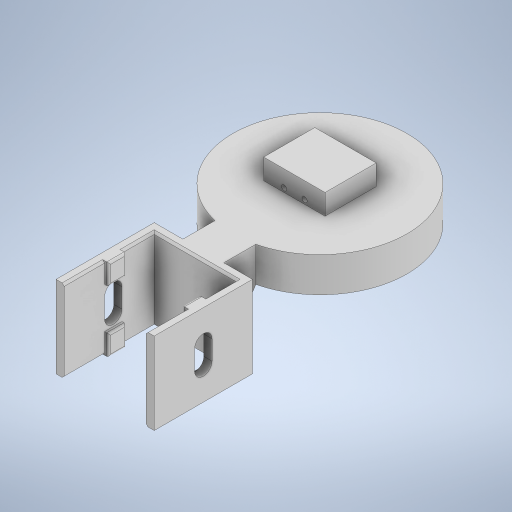
# Autodesk Inventor part: Bi_PAM_top_slot2
Saved by Autodesk Inventor 2024 (Build 280153000, 153)
## iProperties
Created: 2023-07-27
Part Number: Bi_PAM_top_slot2
Material: 일반
Document SubType Name: Modeling
Designer: jsw
Density: 1 g/cm^3
Appearance: 기본값
Author: jsw
Autodesk Inventor part; units mm, degrees
ref_plane "YZ Plane" through (0, 0, 0) normal (1, 0, 0) x (0, 1, 0)
ref_plane "XZ Plane" through (0, 0, 0) normal (0, 1, 0) x (-1, 0, 0)
sketch "스케치1" plane through (0, 0, 0) normal (0, 1, 0) x (-1, 0, 0)
  circle A0 centre (0, 0) radius 39
  circle A1 centre (0, 0) radius 42.5
  dimension "d0" = 78
  dimension "d1" = 3.5
  constraints: 2 centre point, 2 coincident
  measures "d0" diameter of A0
  measures "d1" radial gap between concentric circles of A0 A1
extrude "돌출1" add sketch "스케치1" along normal blind 7 contours A0 | A1
sketch "스케치2" plane through (0, 0, 0) normal (0, -1, 0) x (1, 0, 0)
  line L0 (15, -36.2132) -> (-15, -36.2132)
  line L1 (-15, -36.2132) -> (-36.2132, -15)
  line L2 (-36.2132, -15) -> (-36.2132, 15)
  line L3 (-36.2132, 15) -> (-15, 36.2132)
  line L4 (-15, 36.2132) -> (15, 36.2132)
  line L5 (15, 36.2132) -> (36.2132, 15)
  line L6 (36.2132, 15) -> (36.2132, -15)
  line L7 (36.2132, -15) -> (15, -36.2132)
  point P0 (0, 0)
  point P1 (0, 0)
  dimension "d5" = 30
  constraints: 16 end point, 1 coincident, 1 horizontal, 17 other
  measures "d5" distance of L5.end L6.end
extrude "돌출2" cut sketch "스케치2" against normal blind 4
fillet "모깎기1" radius 1.2 8 edges at (0, 4, 36.2132) (-25.6066, 4, 25.6066) (25.6066, 4, 25.6066) (36.2132, 4, 0) (25.6066, 4, -25.6066) (0, 4, -36.2132) (-25.6066, 4, -25.6066) (-36.2132, 4, 0)
sketch "스케치3" plane through (0, 0, 0) normal (0, -1, 0) x (1, 0, 0)
  line L0 (-15, 36.2132) -> (15, 36.2132) projected
  circle A0 centre (0, 0) radius 39.1969
  circle A1 centre (0, 0) radius 41.1969
  dimension "d9" = 2
  constraints: 2 coincident, 1 centre point, 3 other
extrude "돌출3" cut sketch "스케치3" against normal blind 4
sketch "스케치4" plane through (0, 7, 0) normal (0, 1, 0) x (1, 0, 0)
  line L0 (-15, 12.5) -> (15, 12.5)
  line L1 (15, 12.5) -> (15, -12.5)
  line L2 (15, -12.5) -> (-15, -12.5)
  line L3 (-15, -12.5) -> (-15, 12.5)
  point P0 (0, 0)
  point P1 (0, 12.5)
  point P2 (15, 0)
  dimension "d12" = 30
  dimension "d13" = 25
  constraints: 8 end point, 2 midpoint, 2 parallel, 1 horizontal, 1 horizontal alignment, 1 perpendicular, 1 vertical alignment
  measures "d12" distance of L0.start L0.end
  measures "d13" distance of L0.end L1.end
extrude "돌출4" add sketch "스케치4" along normal blind 10
sketch "스케치10" plane through (0, 0, 0) normal (0, -1, 0) x (1, 0, 0)
  circle A0 centre (0, 0) radius 41.1969 projected
  circle A1 centre (0, 0) radius 42.5 projected
extrude "돌출9" add sketch "스케치10" along normal blind 10
sketch "스케치11" plane through (0, 7, 0) normal (0, 1, 0) x (1, 0, 0)
  line L0 (-10, -61) -> (10, -61)
  line L1 (10, -61) -> (10, -41)
  line L2 (10, -41) -> (-10, -41)
  line L3 (-10, -41) -> (-10, -61)
  line L4 (-10, -61) -> (10, -41) construction
  line L5 (10, -61) -> (-10, -41) construction
  circle A0 centre (0, 0) radius 42.5 projected
  point P0 (0, -51)
  point P1 (10, -41.3068)
  point P2 (-10, -41.3068)
  dimension "d44" = 10
  dimension "d45" = 20
  dimension "d49" = 41
  constraints: 12 end point, 2 midpoint, 2 parallel, 1 horizontal, 1 perpendicular, 1 vertical alignment
  measures "d44" distance from line of point (0, -51) L1
  measures "d45" distance of L0.end L1.end
  measures "d49" distance from line of L2 point (0, 0)
extrude "돌출10" add sketch "스케치11" against normal blind 40 contours L3 A0 L1 L0
sketch "스케치12" plane through (0, 7, 0) normal (0, 1, 0) x (1, 0, 0)
  line L0 (20, -101) -> (-20, -101)
  line L1 (-20, -101) -> (-20, -61)
  line L2 (-20, -61) -> (20, -61)
  line L3 (20, -61) -> (20, -101)
  line L4 (20, -101) -> (-20, -61) construction
  line L5 (-20, -101) -> (20, -61) construction
  line L6 (24, -105) -> (-24, -105)
  line L7 (-24, -105) -> (-24, -57)
  line L8 (-24, -57) -> (24, -57)
  line L9 (24, -57) -> (24, -105)
  line L10 (24, -105) -> (-24, -57) construction
  line L11 (-24, -105) -> (24, -57) construction
  line L12 (-10, -61) -> (10, -61) projected
  line L13 (-20, -101) -> (-20, -105)
  line L14 (20, -101) -> (20, -105)
  point P0 (0, 0)
  point P1 (0, -81)
  point P2 (0, -61)
  dimension "d50" = 40
  dimension "d51" = 40
  dimension "d52" = 4
  dimension "d53" = 20
  constraints: 28 end point, 5 midpoint, 4 parallel, 4 perpendicular, 3 point on line, 2 horizontal, 1 vertical alignment
  measures "d50" distance of L1.end L2.end
  measures "d51" distance of L2.end L0.start
  measures "d52" distance between parallel lines of L2 L8
  measures "d53" distance of point (0, -61) point (0, -81)
extrude "돌출11" add sketch "스케치12" against normal blind 40 contours L3 L2 L1 L13 L6 L7 L8 L9 L14
sketch "스케치13" plane through (-24, 7, 57) normal (-1, 0, 0) x (0, 0, 1)
  line L0 (24, -15.25) -> (24, -24.75) construction
  line L1 (19.75, -15.25) -> (19.75, -24.75)
  line L2 (28.25, -24.75) -> (28.25, -15.25)
  arc A0 (28.25, -15.25) -> (19.75, -15.25) centre (24, -15.25) ccw
  arc A1 (19.75, -24.75) -> (28.25, -24.75) centre (24, -24.75) ccw
  line L3 (0, 0) -> (48, 0) projected
  point P0 (-57, -7)
  point P1 (24, -20)
  point P2 (24, -29)
  point P3 (24, -11)
  point P4 (28.25, -20)
  point P5 (24, 0)
  point P6 (24, 0)
  dimension "d56" = 18
  dimension "d57" = 4.25
  dimension "d58" = 20
  constraints: 8 end point, 6 point on circle, 4 midpoint, 4 tangent, 2 centre point, 1 parallel, 1 vertical, 1 vertical alignment
  measures "d56" distance of point (24, -29) point (24, -11)
  measures "d57" distance of point (24, -20) point (28.25, -20)
  measures "d58" distance of point (24, 0) point (24, -20)
extrude "돌출12" cut sketch "스케치13" against normal up to surface (48 mm away)
sketch "스케치14" plane through (20, 7, 61) normal (-1, 0, 0) x (0, 0, 1)
  line L0 (0, 0) -> (44, 0) projected
  line L1 (15.75, 0) -> (24.25, 0)
  line L2 (24.25, 0) -> (24.25, -10)
  line L3 (24.25, -10) -> (15.75, -10)
  line L4 (15.75, -10) -> (15.75, 0)
  arc A0 (24.25, -15.25) -> (15.75, -15.25) centre (20, -15.25) ccw projected
  line L5 (15.75, -24.75) -> (15.75, -15.25) projected
  line L6 (15.75, -20) -> (24.25, -20)
  line L7 (24.25, -15.25) -> (24.25, -24.75) projected
  line L8 (0, -40) -> (44, -40)
  line L9 (15.75, -40) -> (24.25, -40)
  line L10 (24.25, -40) -> (24.25, -30)
  line L11 (24.25, -30) -> (15.75, -30)
  line L12 (15.75, -30) -> (15.75, -40)
  point P0 (-61, -7)
  point P1 (20, 0)
  point P2 (20, -11)
  point P3 (20, -40)
  point P4 (24.25, -40)
  point P5 (24.25, 0)
  dimension "d61" = 8.5
  dimension "d62" = 10
  constraints: 20 end point, 7 symmetric about line, 3 midpoint, 2 parallel, 2 point on line, 1 horizontal, 1 perpendicular, 1 point on circle, 1 vertical alignment
  measures "d61" distance of L2.end L3.end
  measures "d62" distance of L1.end L2.end
extrude "돌출13" add sketch "스케치14" along normal blind 2 contours L0 L2 L3 L4 | L12 L11 L10 L8
fillet "모깎기2" radius 1 8 edges at (18, 7, 81) (18, 2, 76.75) (18, 2, 85.25) (18, -3, 81) (18, -23, 81) (18, -28, 85.25) (18, -33, 81) (18, -28, 76.75)
ref_plane "작업 평면1" through (0, -33, 105) normal (-1, 0, 0) x (0, 0, 1)
mirror "미러1" about plane through (0, -33, 105) normal (-1, 0, 0) of "모깎기2", "돌출13"
chamfer "모따기2" distance 1 angle 45 10 edges at (20, 7, 68.875) (20, 7, 95.125) (-20, 7, 95.125) (-20, 7, 68.875) (0, 7, 61) (0, -33, 61) (20, -33, 68.875) (20, -33, 95.125) (-20, -33, 95.125) (-20, -33, 68.875)
chamfer "모따기3" distance 15 distance2 23 1 edges at (0, -33, 42.5) measured on face at (0, -33, 43)
sketch "스케치16" plane through (0, 4, 0) normal (0, -1, 0) x (1, 0, 0)
  line L0 (-10.5, -7.75) -> (10.5, -7.75)
  line L1 (10.5, -7.75) -> (10.5, -2.25)
  line L2 (10.5, -2.25) -> (-10.5, -2.25)
  line L3 (-10.5, -2.25) -> (-10.5, -7.75)
  line L4 (-10.5, -7.75) -> (10.5, -2.25) construction
  line L5 (10.5, -7.75) -> (-10.5, -2.25) construction
  line L6 (0, 0) -> (18.5918, 0)
  line L7 (-10.5, 7.75) -> (10.5, 7.75)
  line L8 (10.5, 7.75) -> (10.5, 2.25)
  line L9 (10.5, 2.25) -> (-10.5, 2.25)
  line L10 (-10.5, 2.25) -> (-10.5, 7.75)
  line L11 (-10.5, 7.75) -> (10.5, 2.25) construction
  line L12 (10.5, 7.75) -> (-10.5, 2.25) construction
  point P0 (0, -5)
  point P1 (0, 5)
  dimension "d72" = 21
  dimension "d73" = 5.5
  dimension "d74" = 5
  constraints: 26 end point, 5 symmetric about line, 2 horizontal, 2 midpoint, 2 parallel, 1 perpendicular, 1 vertical alignment
  measures "d72" distance of L2.end L1.end
  measures "d73" distance of L1.end L0.end
  measures "d74" distance from line of L6 point (0, -5)
extrude "돌출14" cut sketch "스케치16" against normal blind 12
chamfer "모따기4" distance 1 angle 45 8 edges at (0, 4, 2.25) (10.5, 4, 5) (0, 4, 7.75) (-10.5, 4, 5) (-10.5, 4, -5) (0, 4, -7.75) (10.5, 4, -5) (0, 4, -2.25)
sketch "스케치17" plane through (15, 7, -12.5) normal (0, 0, -1) x (-1, 0, 0)
  circle A0 centre (20, 2) radius 1.25
  line L0 (26.5, -3) -> (3.5, -3) projected
  line L1 (30, 0) -> (0, 0) projected
  line L2 (15, 0) -> (15, 10)
  line L3 (0, 10) -> (30, 10) projected
  circle A1 centre (10, 2) radius 1.25
  point P0 (15, -7)
  dimension "d80" = 2.5
  dimension "d81" = 5
  dimension "d82" = 10
  constraints: 2 centre point, 2 end point, 2 midpoint, 1 symmetric about line, 1 other
  measures "d80" diameter of A0
  measures "d81" distance from line of L0 A0.centre
  measures "d82" distance of A1.centre A0.centre
extrude "돌출15" cut sketch "스케치17" against normal up to surface (25 mm away)
